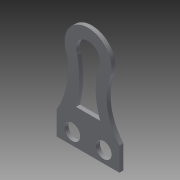
# Autodesk Inventor part: 4-4
Saved by Autodesk Inventor 2015 SP2 (Build 190223200, 223)
## iProperties
Created: 2015-09-21
Part Number: 4-4
Material: Generic
Document SubType Name: Modeling
Designer: KC-019
Density: 1 g/cm^3
Appearance: Default
Author: KC-019
Autodesk Inventor part; units mm, degrees
ref_plane "YZ Plane" through (0, 0, 0) normal (1, 0, 0) x (0, 1, 0)
ref_plane "XZ Plane" through (0, 0, 0) normal (0, 1, 0) x (-1, 0, 0)
ref_plane "XY Plane" through (0, 0, 0) normal (0, 0, 1) x (1, 0, 0)
sketch "Sketch1" plane through (0, 0, 0) normal (0, 0, 1) x (1, 0, 0)
  arc A0 (35.3023, -14.3304) -> (-33.6082, -17.9471) centre (0, 0) ccw
  circle A1 centre (0, 0) radius 19.431
  arc A2 (19.431, 0) -> (19.431, -82.55) centre (138.6611, -41.275) ccw
  arc A3 (-19.431, -82.55) -> (-19.431, 0) centre (-184.2713, -41.275) ccw
  line L0 (-19.431, -82.55) -> (19.431, -82.55)
  arc A4 (35.6836, -13.3526) -> (57.2802, -108.5447) centre (118.9453, -44.5086) ccw
  line L1 (0, -139.7) -> (50.8, -139.7)
  line L2 (50.8, -139.7) -> (50.8, -101.6)
  line L3 (-50.8, -101.6) -> (-50.8, -139.7)
  line L4 (-50.8, -139.7) -> (0, -139.7)
  arc A5 (-50.8, -101.6) -> (-33.6082, -17.9471) centre (-161.9278, -35.1687) ccw
  line L5 (-50.8, -139.7) -> (-25.4, -139.7)
  circle A6 centre (-25.4, -120.65) radius 12.7
  line L6 (50.8, -139.7) -> (25.4, -139.7)
  circle A7 centre (25.4, -120.65) radius 12.7
  dimension "d0" = 76.2
  dimension "d1" = 38.862
  dimension "d5" = 177.8
  dimension "d12" = 101.6
  dimension "d13" = 38.1
  dimension "d14" = 139.7
  dimension "d20" = 25.4
  dimension "d21" = 25.4
  dimension "d23" = 25.4
  constraints: 14 end point, 14 point on circle, 8 centre point, 2 coincident, 2 horizontal, 2 midpoint, 1 perpendicular, 1 point on line, 1 tangent
  measures "d0" diameter of A0
  measures "d1" diameter of A1
  measures "d5" diameter of A4
  measures "d12" distance of L2.end L3.start
  measures "d13" distance of L3.start L3.end
  measures "d14" distance of L1.start point (0, 0)
  measures "d20" diameter of A6
  measures "d21" distance of L1.end L6.end
  measures "d23" diameter of A7
extrude "Extrusion1" add sketch "Sketch1" along normal blind 6.35
body "Solid1"
